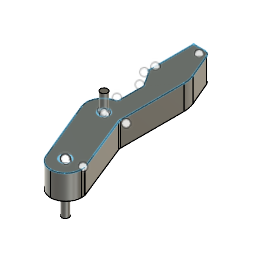
Gripperv3 (Autodesk Fusion 360 archive; units mm, degrees)
design "Part2"
part number: 2026-03-31-11-37-53-286
Autodesk Fusion 360 part; units mm, degrees
sketch "Sketch4" plane through (0, 0, 0) normal (0, 0, 1) x (1, 0, 0)
  line L0 (-5.8, 15.9921) -> (-3.8739, 15.9921)
  line L1 (3.2567, -12.1247) -> (3.2567, -12.6861)
  line L2 (0.5567, -15.3861) -> (0.6374, -15.3861)
  line L3 (-6.1921, -3.2178) -> (-1.8583, -13.7163)
  arc A0 (-1.8583, -13.7163) -> (0.6374, -15.3861) centre (0.6374, -12.6861) ccw
  arc A1 (0.5567, -15.3861) -> (3.2567, -12.6861) centre (0.5567, -12.6861) ccw
  arc A2 (-6.438, -1.9777) -> (-6.1921, -3.2178) centre (-3.188, -1.9777) ccw
  line L4 (-2.9533, 15.3827) -> (-1.1938, 11.2364)
  line L5 (-0.7965, 9.2832) -> (-0.7965, -1.8088)
  line L6 (-0.7242, -2.1821) -> (3.2387, -12.0314)
  arc A3 (3.2567, -12.1247) -> (3.2387, -12.0314) centre (3.0067, -12.1247) ccw
  arc A4 (-0.7965, 9.2832) -> (-1.1938, 11.2364) centre (-5.7965, 9.2832) ccw
  arc A5 (-2.9533, 15.3827) -> (-3.8739, 15.9921) centre (-3.8739, 14.9921) ccw
  arc A6 (-0.7965, -1.8088) -> (-0.7242, -2.1821) centre (0.2035, -1.8088) ccw
  line L7 (-5.4748, 7.788) -> (-3.9887, 5.4995)
  line L8 (-3.9, 5.2) -> (-3.9, 1.2314)
  arc A7 (-5.4748, 7.788) -> (-5.8468, 8.0311) centre (-5.9361, 7.4884) ccw
  arc A8 (-3.9, 5.2) -> (-3.9887, 5.4995) centre (-4.45, 5.2) ccw
  arc A9 (-4.1344, 0.7809) -> (-3.9, 1.2314) centre (-4.45, 1.2314) ccw
  line L9 (-4.1344, 0.7809) -> (-4.8771, 0.4353)
  line L10 (-6.438, -1.9777) -> (-6.438, -2.0126)
  arc A10 (-4.8771, 0.4353) -> (-6.438, -2.0126) centre (-3.738, -2.0126) ccw
  line L11 (-5.851, 15.992) -> (-5.8, 15.9921)
  line L12 (-5.851, 15.992) -> (-5.8468, 8.0311)
  line L13 (-5.851, 15.992) -> (-5.8511, 16.1794)
  line L14 (-5.8511, 16.1794) -> (-6.2056, 16.1792)
  line L15 (-6.2056, 16.1792) -> (-6.2013, 7.9543)
  line L16 (-6.2013, 7.9543) -> (-5.8511, 7.9545)
  line L17 (-5.8511, 7.9545) -> (-5.8468, 8.0311)
  dimension "d9" = 2.7
  dimension "d10" = 3.25
  dimension "d11" = 0.25
  dimension "d12" = 5
  dimension "d13" = 1
  dimension "d14" = 1
  dimension "d15" = 0.55
  dimension "d16" = 2.7
  constraint horizontal L0
  constraint vertical L1
  constraint horizontal L2
  constraint vertical L10
  constraint tangent L3 A0
  constraint tangent L2 A0
  constraint tangent L1 A1
  constraint tangent L2 A1
  constraint equal A0 A1
  constraint tangent L3 A2
  constraint tangent A2 L10
  constraint vertical L5
  constraint tangent L6 A3
  constraint tangent L1 A3
  constraint tangent L4 A4
  constraint tangent L5 A4
  constraint tangent L4 A5
  constraint tangent L0 A5
  constraint tangent L5 A6
  constraint tangent L6 A6
  constraint tangent L7 A7
  constraint tangent L7 A8
  constraint tangent L8 A8
  constraint equal A7 A8
  constraint tangent L8 A9
  constraint equal A7 A9
  constraint tangent L9 A10
  constraint tangent L10 A10
  constraint coincident L11 L12.start
  constraint coincident A7 L12.end
  constraint perpendicular L11 L12
  constraint perpendicular L11 L13
  constraint perpendicular L13 L14
  constraint perpendicular L14 L15
  constraint perpendicular L15 L16
  measures "d9" radius of A0
  measures "d10" radius of A2
  measures "d11" radius of A3
  measures "d12" radius of A4
  measures "d13" radius of A5
  measures "d14" radius of A6
  measures "d15" radius of A7
  measures "d16" radius of A10
extrude "Extrude1" add sketch "Sketch4" along normal blind 4 contours L0 L1 L2 L3 A0 A1 A2 L4 L5 L6 A3 A4 A5 A6 L7 L8 A7 A8 A9 L9 L10 A10 L11 L12
scale "Scale1" factor 2 about (-0.7965, -1.8088, 0) bodies 1
move_face "OffsetFaces1" offset 0.5 1 faces at (-5.0533, -10.9353, 8)
sketch "part2_ext" plane through (0, 0, 8.5) normal (0, 0, 1) x (1, 0, 0)
  arc A0 (-5.1276, 32.5826) -> (-6.9687, 33.8013) centre (-6.9687, 31.8013) ccw
  arc A1 (1.9731, -28.9543) -> (7.2598, -22.9617) centre (1.8924, -23.5549) ccw
  line L0 (7.2598, -22.9617) -> (7.1451, -22.7867)
  arc A2 (-8.9753, 2.6879) -> (-12.0969, -2.1747) centre (-6.697, -2.208) ccw
  arc A3 (-2.9376, -25.6154) -> (1.9731, -28.9543) centre (2.0538, -23.5549) ccw
  line L1 (-1.6086, 24.2899) -> (-5.1276, 32.5826)
  line L2 (-7.021, 12.2172) -> (-7.021, 4.28)
  arc A4 (-0.6695, -2.547) -> (-0.814, -1.8004) centre (1.186, -1.8004) cw
  arc A5 (-7.1985, 12.8163) -> (-7.021, 12.2172) centre (-8.121, 12.2172) cw
  arc A6 (-10.9147, 17.8795) -> (-10.1707, 17.3932) centre (-11.0932, 16.7941) cw
  line L3 (-6.9687, 33.8013) -> (-10.821, 33.8013)
  line L4 (-7.4898, 3.3791) -> (-8.9753, 2.6879)
  arc A7 (-0.814, 20.3836) -> (-1.6086, 24.2899) centre (-10.814, 20.3836) ccw
  line L5 (7.2563, -22.2456) -> (-0.6695, -2.547)
  arc A8 (7.1451, -22.7867) -> (7.2563, -22.2456) centre (6.7924, -22.4322) ccw
  arc A9 (-12.0969, -2.1747) -> (-11.6052, -4.6184) centre (-5.597, -2.1382) ccw
  arc A10 (-7.021, 4.28) -> (-7.4898, 3.3791) centre (-8.121, 4.28) cw
  line L6 (-10.923, 33.8013) -> (-10.9147, 17.8795)
  line L7 (-10.1707, 17.3932) -> (-7.1985, 12.8163)
  line L8 (-11.6052, -4.6184) -> (-2.9376, -25.6154)
  line L9 (-10.821, 33.8013) -> (-10.923, 33.8013)
  line L10 (-0.814, -1.8004) -> (-0.814, 20.3836)
  line L11 (-10.9147, 17.8795) -> (-10.923, 33.8013)
  line L12 (-10.923, 33.8013) -> (-6.9687, 33.8013)
  line L13 (-4.7446, -21.238) -> (-10.2225, -7.9681)
  line L14 (5.125, -16.9486) -> (-0.5508, -2.8419)
  circle A11 centre (1.2992, -23.1297) radius 1.2491
  circle A12 centre (1.2992, -23.1297) radius 1.7482
  circle A13 centre (1.2992, -23.1297) radius 1.2491
  circle A14 centre (1.2992, -23.1297) radius 1.7482
  circle A15 centre (-5.9739, -2.3712) radius 1.2491
  circle A16 centre (-5.9739, -2.3712) radius 1.7482
  point P0 (2.0538, -23.5549)
  point P1 (1.8924, -23.5549)
  point P2 (-5.2192, -2.7964)
  point P3 (-5.3806, -2.7964)
extrude "Extrude2" add sketch "part2_ext" against normal blind 15.03 contours A15
extrude "Extrude3" add sketch "part2_ext" along normal blind 6.53 contours A15
extrude "Extrude4" add sketch "part2_ext" against normal blind 17.15 contours A11 A13
equation "d23 = -8.5 mm - 7.45 mm + 0.92 mm"
equation "d25 = 7.45 mm - 0.92 mm"
equation "d27 = -8.5 mm - 7.45 mm - 1.2 mm"

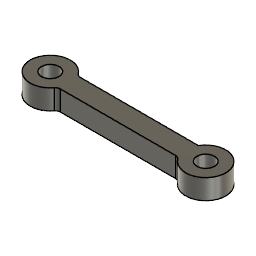
design "Part1"
part number: 2026-03-31-10-29-44-602
Autodesk Fusion 360 part; units mm, degrees
sketch "Sketch1" plane through (0, 0, 0) normal (0, 0, 1) x (1, 0, 0)
  circle A0 centre (0, 0) radius 1.75
  circle A1 centre (-31, 0) radius 1.75
  line L0 (-27, -2) -> (-4, -2)
  line L1 (-27, 2) -> (-3.4641, 2)
  arc A2 (-27.8, 2.4) -> (-27.8, -2.4) centre (-31, 0) ccw
  arc A3 (-3.2, -2.4) -> (-3.4641, 2) centre (0, 0) ccw
  arc A4 (-27, -2) -> (-27.8, -2.4) centre (-27, -3) ccw
  arc A5 (-27.8, 2.4) -> (-27, 2) centre (-27, 3) ccw
  arc A6 (-3.2, -2.4) -> (-4, -2) centre (-4, -3) ccw
  point P0 (-31, 0)
  dimension "d7" = 8
  dimension "d8" = 3.5
  dimension "d9" = 8
  dimension "d10" = 3.5
  dimension "d11" = 1
  dimension "d12" = 1
  dimension "d13" = 1
  constraint coincident A0.centre A3.centre
  constraint concentric A0 A3
  constraint coincident P0 A1.centre
  constraint concentric A1 A2
  constraint horizontal L0
  constraint horizontal L1
  constraint tangent L0 A4
  constraint tangent A2 A4
  constraint tangent L1 A5
  constraint tangent A2 A5
  constraint tangent L0 A6
  constraint tangent A3 A6
  measures "d7" diameter of A3
  measures "d8" diameter of A0
  measures "d9" diameter of A2
  measures "d10" diameter of A1
  measures "d11" radius of A4
  measures "d12" radius of A5
  measures "d13" radius of A6
extrude "Extrude1" add sketch "Sketch1" along normal blind 4
